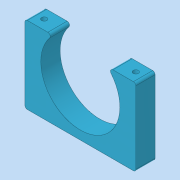
# Autodesk Inventor part: Bottom
Saved by Autodesk Inventor 2017.3 (Build 213256000, 256)
## iProperties
Created: 2018-07-27
Part Number: Bottom
Material: ABS Plastic
Document SubType Name: Modeling
Designer: Derek Wider
Density: 1.06 g/cm^3
Appearance: Turquoise
Author: Derek Wider
Autodesk Inventor part; units mm, degrees
ref_plane "YZ Plane" through (0, 0, 0) normal (1, 0, 0) x (0, 1, 0)
ref_plane "XZ Plane" through (0, 0, 0) normal (0, 1, 0) x (-1, 0, 0)
ref_plane "XY Plane" through (0, 0, 0) normal (0, 0, 1) x (1, 0, 0)
sketch "Sketch1" plane through (0, 0, 0) normal (0, 0, 1) x (1, 0, 0)
  arc A0 (-35.4919, 38.1) -> (35.4919, 38.1) centre (0, 0) ccw
  line L0 (-35.4919, 38.1) -> (-73.025, 38.1)
  line L1 (-73.025, 38.1) -> (-73.025, -63.5)
  line L2 (-73.025, -63.5) -> (73.025, -63.5)
  line L3 (73.025, -63.5) -> (73.025, 38.1)
  line L4 (73.025, 38.1) -> (35.4919, 38.1)
  dimension "d0" = 104.14
  dimension "d1" = 146.05
  dimension "d2" = 101.6
  dimension "d3" = 63.5
  constraints: 10 end point, 3 perpendicular, 2 point on circle, 2 point on line, 1 centre point, 1 coincident, 1 collinear, 1 horizontal
  measures "d0" diameter of A0
  measures "d1" distance between parallel lines of L3 L1
  measures "d2" distance of L0.end L1.end
  measures "d3" distance from line of L2 point (0, 0)
extrude "Extrusion1" add sketch "Sketch1" along normal blind 25.4
sketch "Sketch3" plane through (-73.025, 38.1, 0) normal (0, 1, 0) x (1, 0, 0)
  line L0 (0, 0) -> (37.5331, 0) construction
  line L1 (0, 0) -> (0, -25.4) construction
  line L2 (37.5331, -25.4) -> (0, -25.4) construction
  line L3 (37.5331, 0) -> (37.5331, -25.4) construction
  line L4 (108.5169, 0) -> (146.05, 0) construction
  line L5 (108.5169, 0) -> (108.5169, -25.4) construction
  line L6 (146.05, -25.4) -> (108.5169, -25.4) construction
  line L7 (146.05, 0) -> (146.05, -25.4) construction
  circle A0 centre (12.7, -12.7) radius 3.4925
  circle A1 centre (133.35, -12.7) radius 3.4925
  point P0 (73.025, 0)
  point P1 (0, -12.7)
  dimension "d6" = 6.985
  dimension "d7" = 6.985
  dimension "d8" = 12.7
  dimension "d9" = 12.7
  constraints: 2 centre point, 2 horizontal alignment, 1 midpoint
  measures "d6" diameter of A0
  measures "d7" diameter of A1
  measures "d8" distance from line of A0.centre L1
  measures "d9" distance from line of A1.centre L7
extrude "Extrusion2" cut sketch "Sketch3" against normal blind 25.4
sketch "Sketch4" plane through (0, 0, 0) normal (0, 0, -1) x (-1, 0, 0)
  arc A0 (-35.4919, 38.1) -> (35.4919, 38.1) centre (0, 0) ccw construction
  line L0 (-35.4919, 38.1) -> (-73.025, 38.1) construction
  line L1 (-73.025, 38.1) -> (-73.025, -63.5) construction
  line L2 (-73.025, -63.5) -> (73.025, -63.5) construction
  line L3 (73.025, -63.5) -> (73.025, 38.1) construction
  line L4 (73.025, 38.1) -> (35.4919, 38.1) construction
  line L5 (-66.04, 30.48) -> (-54.61, 30.48)
  line L6 (-54.61, 30.48) -> (-54.61, 24.13)
  line L7 (-54.61, 24.13) -> (-66.04, 24.13)
  line L8 (-66.04, 24.13) -> (-66.04, 30.48)
  line L9 (-60.325, 30.48) -> (-60.325, 24.13) construction
  dimension "d12" = 11.43
  dimension "d13" = 12.7
  dimension "d14" = 7.62
  dimension "d15" = 6.35
  constraints: 10 end point, 2 midpoint, 2 parallel, 1 horizontal, 1 perpendicular
  measures "d12" distance between parallel lines of L6 L8
  measures "d13" distance between parallel lines of L1 L9
  measures "d14" distance between parallel lines of L0 L5
  measures "d15" distance of L7.end L5.start
extrude "Extrusion3" cut sketch "Sketch4" against normal blind 20.32
mirror "Mirror1" about plane through (0, 0, 0) normal (1, 0, 0) of "Extrusion3"
fillet "Fillet1" radius 3.175 6 edges at (-35.4919, 38.1, 12.7) (35.4919, 38.1, 12.7) (-73.025, 38.1, 12.7) (-73.025, -63.5, 12.7) (73.025, -63.5, 12.7) (73.025, 38.1, 12.7)
body "Solid1"
